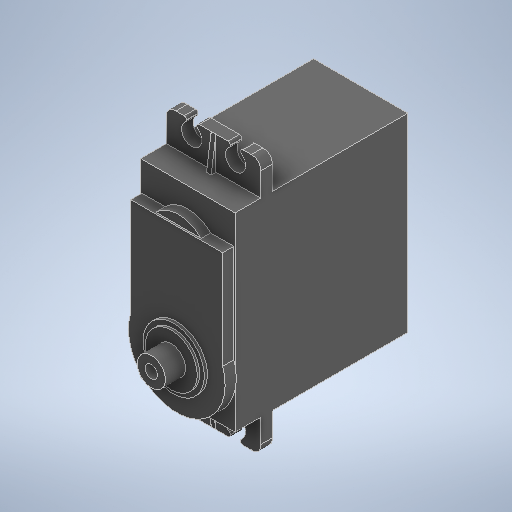
# Autodesk Inventor part: 996R
Saved by Autodesk Inventor 2025.1 (Build 291241000, 241)
## iProperties
Created: 2025-02-24
Part Number: 996R
Material: Generic
Document SubType Name: Modeling
Designer: 13156
Density: 1 g/cm^3
Appearance: Default
Author: 13156
Autodesk Inventor part; units mm, degrees
ref_plane "YZ Plane" through (0, 0, 0) normal (1, 0, 0) x (0, 1, 0)
ref_plane "XZ Plane" through (0, 0, 0) normal (0, 1, 0) x (-1, 0, 0)
ref_plane "XY Plane" through (0, 0, 0) normal (0, 0, 1) x (1, 0, 0)
sketch "Sketch1" plane through (0, 0, 0) normal (0, 0, 1) x (1, 0, 0)
  line L0 (-10, 20.125) -> (10, 20.125)
  line L1 (10, 20.125) -> (10, -20.125)
  line L2 (10, -20.125) -> (-10, -20.125)
  line L3 (-10, -20.125) -> (-10, 20.125)
  line L4 (0, 0) -> (0, 20.8875) construction
  line L5 (0, 0) -> (17.5642, 0) construction
  line L6 (10, 20.125) -> (-10, 20.125)
  line L7 (-10, 20.125) -> (-10, 27.125)
  line L8 (-10, 27.125) -> (10, 27.125)
  line L9 (10, 27.125) -> (10, 20.125)
  line L10 (10, -20.125) -> (-10, -20.125)
  line L11 (-10, -20.125) -> (-10, -27.125)
  line L12 (-10, -27.125) -> (10, -27.125)
  line L13 (10, -27.125) -> (10, -20.125)
  dimension "d0" = 20
  dimension "d1" = 40.25
  dimension "d2" = 7
  constraints: 28 end point, 6 parallel, 4 horizontal, 3 perpendicular, 2 collinear, 1 point on line, 1 vertical, 2 other
  measures "d0" distance of L0.start L0.end
  measures "d1" distance between parallel lines of L2 L0
  measures "d2" distance between parallel lines of L0 L8
extrude "Extrusion1" add sketch "Sketch1" along normal blind 2.45
extrude "Extrusion2" add sketch "Sketch1" along normal blind 7.9 and the other way blind 28.75 contours L0 L1 L2 L3
fillet "Fillet1" radius 2 4 edges at (-10, -27.125, 1.225) (10, -27.125, 1.225) (10, 27.125, 1.225) (-10, 27.125, 1.225) curvature continuous yes
sketch "Sketch2" plane through (0, 0, 2.45) normal (0, 0, 1) x (1, 0, 0)
  circle A0 centre (4.65, -24.425) radius 2.15
  circle A1 centre (-4.65, -24.425) radius 2.15
  circle A2 centre (4.65, 24.425) radius 2.15
  circle A3 centre (-4.65, 24.425) radius 2.15
  line L0 (-10, -20.125) -> (10, -20.125) projected
  line L1 (10, 20.125) -> (-10, 20.125) projected
  line L2 (0, 20.125) -> (0, -31.261) construction
  line L3 (5.75, -26.2723) -> (5.75, -27.125)
  line L4 (5.75, -27.125) -> (3.55, -27.125)
  line L5 (3.55, -27.125) -> (3.55, -26.2723)
  line L6 (-3.55, -26.2723) -> (-3.55, -27.125)
  line L7 (-3.55, -27.125) -> (-5.75, -27.125)
  line L8 (-5.75, -27.125) -> (-5.75, -26.2723)
  line L9 (5.75, 26.2723) -> (5.75, 27.125)
  line L10 (5.75, 27.125) -> (3.55, 27.125)
  line L11 (3.55, 27.125) -> (3.55, 26.2723)
  line L12 (-3.55, 26.2723) -> (-3.55, 27.125)
  line L13 (-5.75, 27.125) -> (-5.75, 26.2723)
  line L14 (8, 27.125) -> (-8, 27.125) projected
  line L15 (-8, -27.125) -> (8, -27.125) projected
  line L16 (-4.65, -24.425) -> (-4.65, -28.2076) construction
  line L17 (4.65, -24.425) -> (4.65, -27.9076) construction
  line L18 (4.65, 24.425) -> (4.65, 28.0006) construction
  line L19 (-4.65, 24.425) -> (-4.65, 28.7991) construction
  line L20 (0.5, -20.125) -> (-0.5, -20.125)
  line L21 (-0.5, -20.125) -> (-0.5, -27.125)
  line L22 (-0.5, -27.125) -> (0.5, -27.125)
  line L23 (0.5, -27.125) -> (0.5, -20.125)
  line L24 (0.5, 20.125) -> (-0.5, 20.125)
  line L25 (-0.5, 20.125) -> (-0.5, 27.125)
  line L26 (-0.5, 27.125) -> (0.5, 27.125)
  line L27 (0.5, 27.125) -> (0.5, 20.125)
  line L28 (0, 20.125) -> (0, 24.1498) construction
  point P0 (0, 0)
  point P1 (-3.55, -26.6986)
  point P2 (5.75, 26.6986)
  point P3 (3.55, 26.6986)
  dimension "d10" = 4.3
  dimension "d11" = 4.3
  dimension "d14" = 4.3
  dimension "d15" = 9.3
  dimension "d16" = 9.3
  dimension "d17" = 2.2
  dimension "d18" = 2.2
  dimension "d23" = 1
  dimension "d24" = 1
  constraints: 50 end point, 16 point on line, 8 point on circle, 7 vertical, 6 perpendicular, 5 parallel, 4 centre point, 4 midpoint, 3 equal radius, 2 collinear, 2 horizontal, 2 symmetric about line, 4 other
  measures "d10" diameter of A0
  measures "d11" distance from line of L0 L17.start
  measures "d14" distance from line of L1 L18.start
  measures "d15" distance of L18.start L19.start
  measures "d16" distance of L16.start L17.start
  measures "d17" distance from line of L8 point (-3.55, -26.699)
  measures "d18" distance of point (5.75, 26.699) point (3.55, 26.699)
  measures "d23" distance between parallel lines of L23 L21
  measures "d24" distance between parallel lines of L25 L27
extrude "Extrusion3" cut sketch "Sketch2" against normal blind 7.9 contours A0 | A0 L3 L4 L5 | A1 | A1 L6 L7 L8 | A2 | A2 L11 L10 L9 | A3 | A3 L13 L14 L12
fillet "Fillet3" radius 0.5 16 edges at (3.55, 26.2723, 1.225) (3.55, 27.125, 1.225) (5.75, 26.2723, 1.225) (5.75, 27.125, 1.225) (-3.55, 26.2723, 1.225) (-3.55, 27.125, 1.225) (-5.75, 27.125, 1.225) (-5.75, 26.2723, 1.225) (-5.75, -26.2723, 1.225) (-5.75, -27.125, 1.225) (3.55, -26.2723, 1.225) (3.55, -27.125, 1.225) (-3.55, -27.125, 1.225) (-3.55, -26.2723, 1.225) (5.75, -27.125, 1.225) (5.75, -26.2723, 1.225) curvature continuous yes
extrude "Extrusion4" add sketch "Sketch2" along normal blind 1 contours L0 L23 L15 L21 | L1 L25 L14 L27
chamfer "Chamfer1" distance 7 distance2 1 1 edges at (0, 27.125, 3.45) measured on face at (0, 26.625, 3.45)
chamfer "Chamfer2" distance 7 distance2 1 1 edges at (0, -27.125, 3.45) measured on face at (0, -26.625, 3.45)
sketch "Sketch3" plane through (0, 0, 7.9) normal (0, 0, 1) x (1, 0, 0)
  circle A0 centre (0, -10.125) radius 9.75
  line L0 (-10, -20.125) -> (10, -20.125) projected
  line L1 (9.75, -10.125) -> (-9.75, -10.125)
  line L2 (-9.75, -10.125) -> (-9.75, 13.875)
  line L3 (-9.75, 13.875) -> (9.75, 13.875)
  line L4 (9.75, 13.875) -> (9.75, -10.125)
  line L5 (-9.75, -10.125) -> (-9.75, -4.0345) construction
  line L6 (-10, 20.125) -> (-10, -20.125) construction
  arc A1 (4.825, 13.875) -> (-4.825, 13.875) centre (0, 9.0548) ccw
  line L7 (10, -20.125) -> (10, 20.125) projected
  circle A2 centre (0, -10.125) radius 10.25
  circle A3 centre (0, -10.125) radius 6.5
  circle A4 centre (0, -10.125) radius 5.5
  circle A5 centre (0, -10.125) radius 3
  circle A6 centre (0, -10.125) radius 1.3
  point P0 (0, 0)
  point P1 (0, 13.875)
  point P2 (0, 15.875)
  point P3 (9.75, -6.9627)
  point P4 (-9.75, -6.9627)
  point P5 (-6.5, -10.125)
  point P6 (6.5, -10.125)
  dimension "d33" = 19.5
  dimension "d34" = 10
  dimension "d35" = 0
  dimension "d36" = 24
  dimension "d37" = 9.65
  dimension "d38" = 2
  dimension "d39" = 0
  dimension "d40" = 0.25
  dimension "d41" = 20.5
  dimension "d42" = 13
  dimension "d43" = 11
  dimension "d44" = 6
  dimension "d45" = 2.6
  constraints: 10 end point, 7 centre point, 5 coincident, 5 point on circle, 3 parallel, 2 midpoint, 2 point on line, 1 horizontal, 1 perpendicular, 1 tangent
  measures "d33" diameter of A0
  measures "d34" distance from line of L0 A0.centre
  measures "d35" distance of L5.start L1.end
  measures "d36" distance from line of L3 point (0, -10.125)
  measures "d37" distance of A1.end A1.start
  measures "d38" distance of point (0, 13.875) point (0, 15.875)
  measures "d39" horizontal distance of point (0, 13.875) point (0, 15.875)
  measures "d40" distance between parallel lines of L7 L4
  measures "d41" diameter of A2
  measures "d42" diameter of A3
  measures "d43" diameter of A4
  measures "d44" diameter of A5
  measures "d45" diameter of A6
extrude "Extrusion5" add sketch "Sketch3" along normal blind 2.35 contours L1 A3 A0 | L4 A2 L7 L0 L2 A0 | A0 L1 A3 | A0 L2 A2 L4 | A3 L1 A4 | L1 A4 A3 | A2 L2 L3 L4 | A4 L1 A5 | L1 A5 A4 | A2 L7 | L0 A2 | A5 L1 A6 | L1 A6 A5 | A6 L1 | L1 A6
extrude "Extrusion6" add sketch "Sketch3" along normal blind 2 contours L3 A1
extrude "Extrusion7" add sketch "Sketch3" along normal blind 3 contours A3 L1 A4 | L1 A4 A3 | A4 L1 A5 | L1 A5 A4 | A5 L1 A6 | L1 A6 A5 | A6 L1 | L1 A6
extrude "Extrusion8" add sketch "Sketch3" along normal blind 3.5 contours A4 L1 A5 | L1 A5 A4 | A5 L1 A6 | L1 A6 A5 | A6 L1 | L1 A6
extrude "Extrusion9" add sketch "Sketch3" along normal blind 7.75 contours A5 L1 A6 | L1 A6 A5
sketch "Sketch4" plane through (-10, -20.125, 0) normal (0, -1, 0) x (1, 0, 0)
  line L0 (14, -25.75) -> (6, -25.75)
  line L1 (6, -25.75) -> (6, -21.25)
  line L2 (6, -21.25) -> (14, -21.25)
  line L3 (14, -21.25) -> (14, -25.75)
  line L4 (0, -28.75) -> (20, -28.75) construction
  line L5 (10, -28.75) -> (10, -6.1865) construction
  point P0 (10, 0)
  point P1 (10, -21.25)
  dimension "d56" = 8
  dimension "d57" = 4.5
  dimension "d58" = 3
  constraints: 10 end point, 2 midpoint, 2 parallel, 1 horizontal, 1 perpendicular, 1 vertical, 1 other
  measures "d56" distance of L0.start L0.end
  measures "d57" distance from line of point (10, -21.25) L0
  measures "d58" distance between parallel lines of L0 L4
extrude "Extrusion10" add sketch "Sketch4" along normal blind 5.25
chamfer "Chamfer3" distance 1 distance2 5.25 2 edges at (0, -25.375, -21.25) (0, -25.375, -25.75) measured on face at (0, -25.375, -21.75) measured on face at (0, -25.375, -25.25)
chamfer "Chamfer4" distance 1 distance2 5.25 1 edges at (4, -25.375, -23.5) measured on face at (3.5, -25.375, -23.5)
chamfer "Chamfer5" distance 1 distance2 5.25 1 edges at (-4, -25.375, -23.5) measured on face at (-3.5, -25.375, -23.5)
equation "\"d14\" = d11"
equation "\"d15\" = d16"
equation "\"d18\" = d17"
equation "\"d23\" = d24"
body "Solid1"
